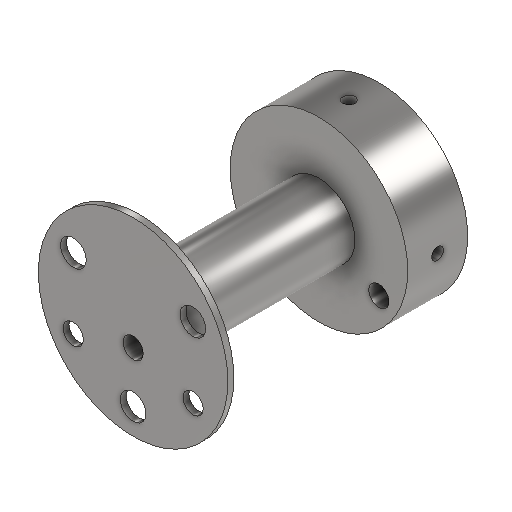
# Autodesk Inventor part: B_pipe_cylinder_5_1
Saved by Autodesk Inventor 2026.2 (Build 302298000, 298)
## iProperties
Created: 2026-02-02
Part Number: B_pipe_cylinder_5_1
Material: ステンレス鋼 440C
Document SubType Name: Modeling
Designer: zetsu
Density: 7.75 g/cm^3
Appearance: 半つや出し
Author: zetsu
Autodesk Inventor part; units mm, degrees
sketch "スケッチ2" plane through (0, 0, 0) normal (0, 0, 1) x (1, 0, 0)
  circle A0 centre (0, 0) radius 15.8
  dimension "d0" = 31.6
  constraints: 1 centre point, 1 coincident
  measures "d0" diameter of A0
extrude "押し出し1" add sketch "スケッチ2" against normal blind 1
sketch "スケッチ11" plane through (0, 0, -1) normal (0, 0, -1) x (-1, 0, 0)
  circle A0 centre (0, 0) radius 6
  dimension "d85" = 12
  constraints: 1 centre point, 1 coincident
  measures "d85" diameter of A0
extrude "押し出し9" add sketch "スケッチ11" along normal blind 30
sketch "スケッチ12" plane through (0, 0, -31) normal (0, 0, -1) x (-1, 0, 0)
  circle A0 centre (0, 0) radius 14.8
  dimension "d106" = 29.6
  constraints: 1 centre point, 1 coincident
  measures "d106" diameter of A0
extrude "押し出し10" add sketch "スケッチ12" along normal blind 10
sketch "スケッチ13" plane through (0, 0, 0) normal (0, 0, 1) x (1, 0, 0)
  circle A0 centre (0, -3) radius 1.7
  circle A1 centre (-10, -6) radius 1.7
  circle A2 centre (10, -6) radius 1.7
  line L0 (0, 0) -> (0, 17.9574) construction
  dimension "d90" = 3.4
  dimension "d91" = 3.4
  dimension "d92" = 3.4
  dimension "d93" = 3
  dimension "d94" = 6
  dimension "d95" = 10
  constraints: 3 centre point, 2 end point, 1 symmetric about line, 1 vertical
  measures "d90" diameter of A0
  measures "d91" diameter of A1
  measures "d92" diameter of A2
  measures "d93" distance of L0.start A0.centre
  measures "d94" vertical distance of A2.centre L0.start
  measures "d95" horizontal distance of A2.centre L0.start
extrude "押し出し11" cut sketch "スケッチ13" against normal through all
sketch "スケッチ14" plane through (0, 0, 0) normal (0, 0, 1) x (1, 0, 0)
  circle A0 centre (0, -11.5) radius 2.15
  circle A1 centre (9.9593, 5.75) radius 2.15
  circle A2 centre (-9.9593, 5.75) radius 2.15
  point P0 (0, 0)
  dimension "d98" = 4.3
  dimension "d99" = 11.5
  dimension "d102" = 360
  constraints: 3 centre point, 7 other
  measures "d98" diameter of A0
  measures "d99" distance of A0.centre point (0, 0)
extrude "押し出し12" cut sketch "スケッチ14" against normal blind 1
ref_plane "作業平面1" through (15, 0, 0) normal (1, 0, 0) x (0, 1, 0)
ref_plane "作業平面2" through (-15, 0, 0) normal (1, 0, 0) x (0, 1, 0)
ref_plane "作業平面3" through (0, 15, 0) normal (0, 1, 0) x (-1, 0, 0)
ref_plane "作業平面4" through (0, -15, 0) normal (0, 1, 0) x (-1, 0, 0)
sketch "スケッチ16" plane through (15, 0, 0) normal (1, 0, 0) x (0, 1, 0)
  circle A0 centre (0, -36) radius 1
  line L0 (-14.8, -41) -> (14.8, -41) projected
  point P0 (0, 0)
  dimension "d111" = 2
  dimension "d112" = 5
  constraints: 1 centre point
  measures "d111" diameter of A0
  measures "d112" distance from line of L0 A0.centre
sketch "スケッチ17" plane through (0, 15, 0) normal (0, 1, 0) x (-1, 0, 0)
  circle A0 centre (0, -36) radius 1
  line L0 (-14.8, -41) -> (14.8, -41) projected
  point P0 (0, 0)
  dimension "d113" = 2
  dimension "d114" = 5
  constraints: 1 centre point
  measures "d113" diameter of A0
  measures "d114" distance from line of A0.centre L0
sketch "スケッチ18" plane through (-15, 0, 0) normal (1, 0, 0) x (0, 1, 0)
  circle A0 centre (0, -36) radius 1
  line L0 (-14.8, -41) -> (14.8, -41) projected
  point P0 (0, 0)
  dimension "d115" = 2
  dimension "d116" = 5
  constraints: 1 centre point
  measures "d115" diameter of A0
  measures "d116" distance from line of L0 A0.centre
sketch "スケッチ19" plane through (0, -15, 0) normal (0, 1, 0) x (-1, 0, 0)
  circle A0 centre (0, -36) radius 1
  line L0 (-14.8, -41) -> (14.8, -41) projected
  point P0 (0, 0)
  dimension "d117" = 2
  dimension "d118" = 5
  constraints: 1 centre point
  measures "d117" diameter of A0
  measures "d118" distance from line of L0 A0.centre
extrude "押し出し13" cut sketch "スケッチ16" against normal blind 5
extrude "押し出し14" cut sketch "スケッチ17" against normal blind 5
extrude "押し出し15" cut sketch "スケッチ18" along normal blind 5
extrude "押し出し16" cut sketch "スケッチ19" along normal blind 5
